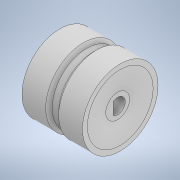
# Autodesk Inventor part: koło
Saved by Autodesk Inventor 2022 (Build 260153000, 153)
## iProperties
Created: 2022-05-14
Part Number: koło
Material: Generic
Document SubType Name: Modeling
Designer: Kamil
Density: 1 g/cm^3
Appearance: Default
Author: Kamil
Autodesk Inventor part; units mm, degrees
ref_plane "YZ Plane" through (0, 0, 0) normal (1, 0, 0) x (0, 1, 0)
ref_plane "XZ Plane" through (0, 0, 0) normal (0, 1, 0) x (-1, 0, 0)
ref_plane "XY Plane" through (0, 0, 0) normal (0, 0, 1) x (1, 0, 0)
sketch "Sketch1" plane through (0, 0, 0) normal (0, 1, 0) x (-1, 0, 0)
  line L0 (0, 0) -> (14, 0)
  line L1 (14, 0) -> (14, -8.75)
  line L2 (14, -8.75) -> (0, -8.75)
  line L3 (0, -8.75) -> (0, 0)
  line L4 (14, 0) -> (0, 0)
  line L5 (0, 0) -> (0, -8)
  line L6 (0, -8) -> (14, -8)
  line L7 (14, -8) -> (14, 0)
  line L8 (0, -8.75) -> (5.5, -8.75)
  line L9 (14, -8.75) -> (8.5, -8.75)
  line L10 (8.5, -8.75) -> (8.5, -4)
  line L11 (5.5, -8.75) -> (5.5, -4)
  line L12 (5.5, -8) -> (7, -8)
  line L13 (5.5, -8) -> (6.25, -8)
  line L14 (8.5, -8) -> (7, -8)
  line L15 (8.5, -8) -> (7.75, -8)
  line L16 (7.75, -8) -> (8.5, -8.75)
  line L17 (6.25, -8) -> (5.5, -8.75)
  dimension "d0" = 14
  dimension "d1" = 8.75
  dimension "d2" = 8
  dimension "d3" = 5.5
  dimension "d4" = 5.5
  constraints: 36 end point, 8 point on line, 4 parallel, 4 perpendicular, 3 midpoint, 2 horizontal, 1 collinear, 1 vertical
  measures "d0" distance of L1.end L2.end
  measures "d1" distance of L0.end L1.end
  measures "d2" distance of L5.end L4.end
  measures "d3" distance of L2.end L8.end
  measures "d4" distance of L1.end L9.end
revolve "Revolution1" add sketch "Sketch1" angle 360 about axis through (0, 0, 0) along (-1, 0, 0) contours L0 L1 L6 L3 | L6 L11 L2 L3 | L1 L2 L10 L6 | L6 L17 L11 | L10 L16 L6
sketch "Sketch2" plane through (0, 0, 0) normal (1, 0, 0) x (0, 0, -1)
  circle A0 centre (0, 0) radius 1.5
  line L0 (-1.5, 0) -> (-1, 0)
  line L1 (-1, 0) -> (-1, 1.118)
  line L2 (-1, 0) -> (-1, -1.118)
  circle A1 centre (0, 0) radius 2.75
  dimension "d6" = 3
  dimension "d7" = 0.5
  dimension "d8" = 5.5
  constraints: 6 end point, 3 point on circle, 2 centre point, 2 coincident, 1 horizontal, 1 perpendicular, 1 point on line
  measures "d6" diameter of A0
  measures "d7" distance of L0.start L0.end
  measures "d8" diameter of A1
extrude "Extrusion1" cut sketch "Sketch2" against normal blind 10 contours A0 L2 L1
extrude "Extrusion2" cut sketch "Sketch2" against normal blind 0.6 contours L1 L0 A0 | A0 L0 L2 | A1
fillet "Fillet1" radius 20 1 edges at (0, 0, 2.75)
sketch "Sketch3" plane through (-14, 0, 0) normal (-1, 0, 0) x (0, 0, 1)
  circle A0 centre (0, 0) radius 8.75 projected
  line L0 (0, -8.75) -> (0, -6.75)
  line L1 (0, 8.75) -> (0, 6.75)
  circle A1 centre (0, 0) radius 6.75
  dimension "d14" = 2
  dimension "d15" = 2
  constraints: 4 end point, 2 point on circle, 2 vertical, 1 coincident, 1 vertical alignment, 2 other
  measures "d14" distance of L0.start L0.end
  measures "d15" distance of L1.start L1.end
extrude "Extrusion3" cut sketch "Sketch3" against normal blind 1 contours A1
fillet "Fillet2" radius 0.5 1 edges at (-14, 0, -6.75)
sketch "Sketch4" plane through (-0.6, 0, 0) normal (1, 0, 0) x (0, 0, -1)
  circle A0 centre (0, 0) radius 2.75 projected
  line L0 (-1, 1.118) -> (-1, -1.118) projected
  arc A1 (-1, -1.118) -> (-1, 1.118) centre (0, 0) ccw projected
  line L1 (1.5, 0) -> (1.6492, 0)
  line L2 (1.5, 0) -> (1.75, 0)
  circle A2 centre (0, 0) radius 1.75
  line L3 (-1, 1.118) -> (-1, -1.118) projected
  line L4 (-1, 0) -> (-1.25, 0)
  line L5 (-1.25, 0) -> (-1.25, 1.2247)
  line L6 (-1.25, 0) -> (-1.25, -1.2247)
  dimension "d19" = 0.25
  dimension "d20" = 0.25
  constraints: 10 end point, 4 point on circle, 3 horizontal, 1 centre point, 1 coincident, 1 midpoint, 1 point on line, 1 vertical
  measures "d19" distance of L1.start L2.end
  measures "d20" distance of L4.start L4.end
extrude "Extrusion4" cut sketch "Sketch4" against normal blind 9.4 contours L0 L4 L5 A2 L2 L1 A1 | L0 A1 L1 L2 A2 L6 L4
sketch "Sketch5" plane through (-14, 0, 0) normal (-1, 0, 0) x (0, 0, 1)
  circle A0 centre (0, 0) radius 8.75 projected
  circle A1 centre (0, 0) radius 7.25 projected
  circle A2 centre (0, 0) radius 8.75
  constraints: 1 centre point, 1 coincident, 1 concentric
extrude "Extrusion5" add sketch "Sketch5" against normal blind 1 contours A0 | A1
sketch "Sketch6" plane through (-0.6, 0, 0) normal (1, 0, 0) x (0, 0, -1)
  arc A0 (-1.25, -1.2247) -> (-1.25, 1.2247) centre (0, 0) ccw projected
  line L0 (-1.25, -1.2247) -> (-1.25, 1.2247) projected
  circle A1 centre (0, 0) radius 2.75 projected
  circle A2 centre (0, 0) radius 1.75
  line L1 (-1.25, -1.2247) -> (-1.25, 1.2247) projected
  line L2 (-1.25, 0) -> (-1, 0)
  line L3 (-1, 0) -> (-1, -1.4361)
  arc A3 (-1.25, -1.2247) -> (-1.25, 1.2247) centre (0, 0) ccw projected
  line L4 (-1, 0) -> (-1, 1.4361)
  dimension "d25" = 0.25
  constraints: 6 end point, 2 point on circle, 1 centre point, 1 coincident, 1 horizontal, 1 midpoint, 1 perpendicular, 1 point on line
  measures "d25" distance of L2.start L2.end
extrude "Extrusion6" add sketch "Sketch6" against normal blind 10 contours L0 L2 L3 A0 | L0 A0 L4 L2
body "Solid1"
